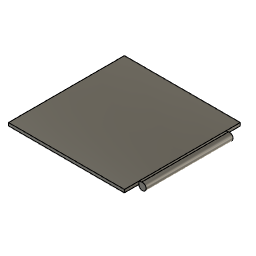
final monetki (Autodesk Fusion 360 archive; units mm, degrees)
design "krishka"
Autodesk Fusion 360 part; units mm, degrees
sketch "Sketch1" plane through (0, 0, 0) normal (0, 0, 1) x (1, 0, 0)
  line L0 (-80, 80) -> (80, 80)
  line L1 (80, 80) -> (80, -80)
  line L2 (80, -80) -> (-80, -80)
  line L3 (-80, -80) -> (-80, 80)
  line L4 (-80, 80) -> (80, -80) construction
  line L5 (80, 80) -> (-80, -80) construction
  dimension "d1" = 160
  dimension "d2" = 160
  constraint horizontal L0
  constraint perpendicular L0 L1
  constraint parallel L0 L2
  constraint parallel L1 L3
  constraint coincident L4 origin
  constraint coincident L5 origin
  measures "d1" distance of L0.start L2.end
  measures "d2" distance of L0.start L0.end
extrude "Extrude1" add sketch "Sketch1" along normal blind 4
ref_plane "WorkPlane1" through (0, -60, 2) normal (0, -1, 0) x (1, 0, 0)
sketch "Sketch2" plane through (0, -60, 2) normal (0, -1, 0) x (1, 0, 0)
  line L0 (80, -2) -> (119, -2) construction
  line L1 (80, 2) -> (83.9024, 2.878)
  arc A0 (80, -2) -> (83.9024, 2.878) centre (85, -2) ccw
  line L2 (80, 2) -> (80, -2)
  point P0 (-80, -2)
  point P1 (-80, 2)
  dimension "d6" = 10
  dimension "d7" = 4
  dimension "d8" = 160
  dimension "d9" = 160
  constraint horizontal L0
  constraint coincident L0 A0.centre
  constraint tangent L1 A0
  measures "d6" diameter of A0
  measures "d7" distance of L0.start L1.start
  measures "d8" distance of L0.start P0
  measures "d9" distance of L1.start P1
extrude "Extrude2" add sketch "Sketch2" against normal blind 120
